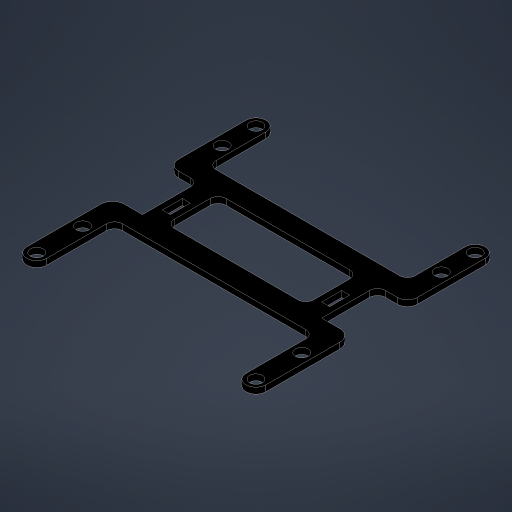
# Autodesk Inventor part: HandleHolder_V2-Carbon
Saved by Autodesk Inventor 2023 (Build 270158000, 158)
## iProperties
Created: 2023-04-10
Part Number: HandleHolder_V2-Carbon
Material: Generic
Document SubType Name: Modeling
Designer: Elias Braun
Density: 1 g/cm^3
Appearance: Default
Author: Elias Braun
Autodesk Inventor part; units mm, degrees
ref_plane "YZ Plane" through (0, 0, 0) normal (1, 0, 0) x (0, 1, 0)
ref_plane "XZ Plane" through (0, 0, 0) normal (0, 1, 0) x (-1, 0, 0)
ref_plane "XY Plane" through (0, 0, 0) normal (0, 0, 1) x (1, 0, 0)
sketch "Sketch1" plane through (0, 0, 0) normal (0, 1, 0) x (-1, 0, 0)
  line L0 (0, 0) -> (0, -5.5344) construction
  line L1 (0, 0) -> (-3.3399, 0) construction
  arc A0 (27.5, 8) -> (30, 10.5) centre (27.5, 10.5) ccw
  arc A1 (-30, 10.5) -> (-27.5, 8) centre (-27.5, 10.5) ccw
  line L2 (25, 13) -> (-25, 13)
  line L3 (22.5, 8) -> (27.5, 8)
  line L4 (-27.5, 8) -> (-22.5, 8)
  line L5 (21, 2.5) -> (21, -2.5)
  line L6 (21, -2.5) -> (19, -2.5)
  line L7 (19, -2.5) -> (19, 2.5)
  line L8 (19, 2.5) -> (21, 2.5)
  line L9 (21, 2.5) -> (19, -2.5) construction
  line L10 (21, -2.5) -> (19, 2.5) construction
  line L11 (-17.5, 0) -> (-20, 0) construction
  line L12 (-19, 2.5) -> (-19, -2.5)
  line L13 (-19, -2.5) -> (-21, -2.5)
  line L14 (-21, -2.5) -> (-21, 2.5)
  line L15 (-21, 2.5) -> (-19, 2.5)
  line L16 (-19, 2.5) -> (-21, -2.5) construction
  line L17 (-19, -2.5) -> (-21, 2.5) construction
  line L18 (17.5, 8) -> (-17.5, 8)
  line L19 (17.5, 8) -> (-17.5, 8)
  circle A2 centre (27.5, 27.5) radius 1.6
  circle A3 centre (-27.5, 27.5) radius 1.6
  line L20 (0, 0) -> (0, 8) construction
  arc A4 (30, 27.5) -> (25, 27.5) centre (27.5, 27.5) ccw
  line L21 (30, 27.5) -> (30, 10.5)
  line L22 (25, 13) -> (25, 27.5)
  arc A5 (-25, 27.5) -> (-30, 27.5) centre (-27.5, 27.5) ccw
  line L23 (-30, 27.5) -> (-30, 10.5)
  line L24 (-25, 13) -> (-25, 27.5)
  line L25 (27.5, 27.5) -> (27.5, 16) construction
  circle A6 centre (27.5, 16) radius 1.6
  circle A7 centre (-27.5, 16) radius 1.6
  arc A8 (30, -10.5) -> (27.5, -8) centre (27.5, -10.5) ccw
  arc A9 (-27.5, -8) -> (-30, -10.5) centre (-27.5, -10.5) ccw
  line L26 (25, -13) -> (-25, -13)
  line L27 (22.5, -8) -> (27.5, -8)
  line L28 (-27.5, -8) -> (-22.5, -8)
  line L29 (17.5, -8) -> (-17.5, -8)
  line L30 (17.5, -8) -> (-17.5, -8)
  circle A10 centre (27.5, -27.5) radius 1.6
  circle A11 centre (-27.5, -27.5) radius 1.6
  arc A12 (25, -27.5) -> (30, -27.5) centre (27.5, -27.5) ccw
  line L31 (30, -27.5) -> (30, -10.5)
  line L32 (25, -13) -> (25, -27.5)
  line L33 (-25, -13) -> (-25, -27.5)
  line L34 (-30, -27.5) -> (-30, -10.5)
  arc A13 (-30, -27.5) -> (-25, -27.5) centre (-27.5, -27.5) ccw
  circle A14 centre (27.5, -16) radius 1.6
  circle A15 centre (-27.5, -16) radius 1.6
  line L35 (22.5, -8) -> (22.5, 8)
  line L36 (17.5, 8) -> (17.5, -8)
  line L37 (-17.5, -8) -> (-17.5, 8)
  line L38 (-22.5, 8) -> (-22.5, -8)
  line L39 (27.5, -16) -> (27.5, -19)
  circle A16 centre (27.5, -19) radius 1.6
  circle A17 centre (-27.5, -19) radius 1.6
  point P0 (20, 0)
  point P1 (0, -8)
  dimension "d16" = 5
  dimension "d17" = 2
  dimension "d18" = 2.5
  dimension "d19" = 5
  dimension "d20" = 2
  dimension "d41" = 8
  dimension "d44" = 11.5
  dimension "d45" = 3.2
  dimension "d66" = 3
  dimension "d67" = 3.2
  constraints: 80 end point, 29 symmetric about line, 18 centre point, 16 point on circle, 9 vertical, 7 parallel, 4 midpoint, 2 coincident, 2 horizontal, 2 perpendicular, 11 other
  measures "d16" distance of L5.start L5.end
  measures "d17" distance of L5.end L6.end
  measures "d18" distance of L11.start L11.end
  measures "d19" distance of L12.start L12.end
  measures "d20" distance of L12.end L13.end
  measures "d41" distance of L0.start L20.end
  measures "d44" distance of L25.start L25.end
  measures "d45" diameter of A6
  measures "d66" distance of L39.start L39.end
  measures "d67" diameter of A16
extrude "Extrusion1" add sketch "Sketch1" along normal blind 1.5 contours L3 L35 L27 A8 L31 A12 L32 L26 L33 A13 L34 A9 L28 L38 L4 A1 L23 A5 L24 L2 L22 A4 L21 A0 | A14 A16 | A15 A17 picked at (27.4973, -15.4078) picked at (-27.5657, -15.4115)
fillet "Fillet1" radius 2 6 edges at (22.5, 0.75, 8) (-22.5, 0.75, 8) (-17.5, 0.75, 8) (17.5, 0.75, 8) (-25, 0.75, 13) (25, 0.75, 13)
sketch "Sketch5" plane through (0, 1.5, 0) normal (0, 1, 0) x (1, 0, 0)
  arc A0 (-23, -13) -> (-25, -15) centre (-23, -15) ccw projected
  line L0 (-25, -15) -> (25, -15)
  line L1 (25, -15) -> (25, -10.5)
  line L2 (25, -10.5) -> (-25, -10.5)
  line L3 (-25, -10.5) -> (-25, -15)
  arc A1 (-17.5, -6) -> (-15.5, -8) centre (-15.5, -6) ccw projected
  line L4 (-17.5, -6) -> (17.5, -6)
  line L5 (17.5, -6) -> (17.5, -8)
  line L6 (17.5, -8) -> (-17.5, -8)
  line L7 (-17.5, -8) -> (-17.5, -6)
  line L8 (-17.5, -6) -> (17.5, -6)
  line L9 (17.5, -6) -> (17.5, -5)
  line L10 (17.5, -5) -> (-17.5, -5)
  line L11 (-17.5, -5) -> (-17.5, -6)
  line L12 (-17.5, 16.5) -> (17.5, 16.5)
  line L13 (17.5, 16.5) -> (17.5, 18.5)
  line L14 (17.5, 18.5) -> (-17.5, 18.5)
  line L15 (-17.5, 18.5) -> (-17.5, 16.5)
  point P0 (0, 0)
  point P1 (17.5, -6)
  dimension "d49" = 50
  dimension "d50" = 4.5
  dimension "d56" = 2
  dimension "d57" = 35
  dimension "d58" = 1
  dimension "d59" = 35
  dimension "d60" = 2
  constraints: 32 end point, 8 parallel, 4 horizontal, 4 perpendicular
  measures "d49" distance of L2.end L1.end
  measures "d50" distance of L1.end L0.end
  measures "d56" distance of L4.end L5.end
  measures "d57" distance of L10.end L9.end
  measures "d58" distance of L9.end L8.end
  measures "d59" distance of L14.end L13.end
  measures "d60" distance of L13.end L12.end
extrude "Extrusion6" cut sketch "Sketch5" against normal blind 1.5 contours L3 L2 L1 L0
extrude "Extrusion7" add sketch "Sketch5" against normal blind 1.5 contours L4 L5 L6 A1 | L11 L10 L9 L4 | A1 L6 L7
fillet "Fillet5" radius 2 10 edges at (-25, 0.75, 10.5) (25, 0.75, 10.5) (22.5, 0.75, -8) (17.5, 0.75, -8) (17.5, 0.75, 5) (-17.5, 0.75, 5) (-17.5, 0.75, -8) (-22.5, 0.75, -8) (25, 0.75, -13) (-25, 0.75, -13)
sketch "Sketch6" plane through (0, 1.5, 0) normal (0, 1, 0) x (1, 0, 0)
  line L0 (-30, -10.5) -> (-30, -27.5) projected
  arc A0 (-24.5, -8) -> (-22.5, -6) centre (-24.5, -6) ccw projected
  line L1 (-30, -10.5) -> (-22.5, -10.5)
  line L2 (-22.5, -10.5) -> (-22.5, -6)
  line L3 (-22.5, -6) -> (-30, -6)
  line L4 (-30, -6) -> (-30, -10.5)
  line L5 (30, -27.5) -> (30, -10.5) projected
  line L6 (22.4338, -6) -> (30, -6)
  line L7 (30, -6) -> (30, -10.5)
  line L8 (30, -10.5) -> (22.4338, -10.5)
  line L9 (22.4338, -10.5) -> (22.4338, -6)
  arc A1 (27.5, 18.5) -> (30, 21) centre (27.5, 21) ccw projected
  arc A2 (24.5, 18.5) -> (22.5, 16.5) centre (24.5, 16.5) ccw projected
  line L10 (30, 21) -> (22.5, 21)
  line L11 (22.5, 21) -> (22.5, 16.5)
  line L12 (22.5, 16.5) -> (30, 16.5)
  line L13 (30, 16.5) -> (30, 21)
  arc A3 (-30, 21) -> (-27.5, 18.5) centre (-27.5, 21) ccw projected
  line L14 (-30, 21) -> (-22.5, 21)
  line L15 (-22.5, 21) -> (-22.5, 16.5)
  line L16 (-22.5, 16.5) -> (-30, 16.5)
  line L17 (-30, 16.5) -> (-30, 21)
  point P0 (0, 0)
  constraints: 32 end point, 8 parallel, 4 horizontal, 4 perpendicular, 3 point on line
extrude "Extrusion8" add sketch "Sketch6" against normal blind 1.5 contours L4 L3 L2 L1 | L6 L7 L8 L9
fillet "Fillet6" radius 3 2 edges at (30, 0.75, 6) (-30, 0.75, 6)
body "Solid1"
